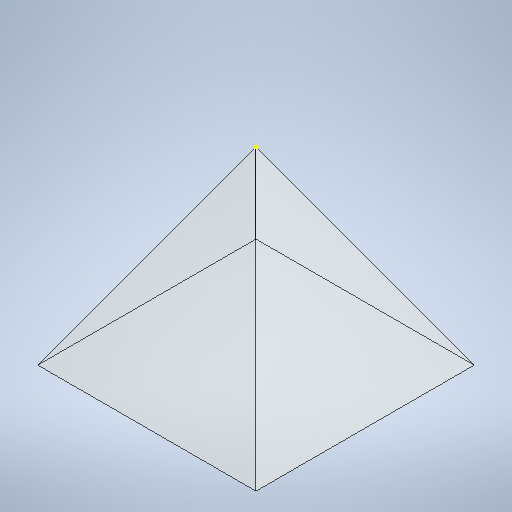
# Autodesk Inventor part: vl53l7cx-FOV
Saved by Autodesk Inventor 2025 (Build 290162000, 162)
## iProperties
Created: 2026-03-19
Part Number: vl53l7cx-FOV
Material: Glass
Document SubType Name: Modeling
Designer: steve
Density: 2.18 g/cm^3
Appearance: Clear
Author: steve
Autodesk Inventor part; units mm, degrees
ref_plane "YZ Plane" through (0, 0, 0) normal (1, 0, 0) x (0, 1, 0)
ref_plane "XZ Plane" through (0, 0, 0) normal (0, 1, 0) x (-1, 0, 0)
sketch "Sketch1" plane through (0, 0, 0) normal (0, 0, 1) x (1, 0, 0)
  line L0 (0, 200) -> (0, -1200) construction
  line L1 (-808.2904, 0) -> (808.2904, 0) construction
  line L2 (0, 0) -> (-577.3503, -1000)
  line L3 (-577.3503, -1000) -> (577.3503, -1000)
  line L4 (577.3503, -1000) -> (0, 0)
  point P0 (0, -1000)
  dimension "d0" = 60
  dimension "d1" = 1000
  constraints: 6 end point, 1 horizontal, 1 midpoint, 1 point on line
  measures "d0" angle of L4 L2
  measures "d1" distance from line of L2.start L3
sketch "Sketch2" plane through (0, 0, 0) normal (1, 0, 0) x (0, 1, 0)
  line L0 (0, 0) -> (-1000, 577.3503)
  line L1 (-1000, 577.3503) -> (-1000, -577.3503)
  line L2 (-1000, -577.3503) -> (0, 0)
  line L3 (0, 677.3503) -> (-1000, 677.3503)
  line L4 (-1000, 677.3503) -> (-1000, -677.3503)
  line L5 (-1000, -677.3503) -> (0, -677.3503)
  line L6 (0, -677.3503) -> (0, 677.3503)
  point P0 (-1000, 0)
  point P1 (-1000, 0)
  point P2 (-1000, 0)
  point P3 (-1000, 0)
  dimension "d2" = 60
  dimension "d4" = 100
  constraints: 14 end point, 2 midpoint, 2 parallel, 1 coincident, 1 collinear, 1 horizontal, 1 perpendicular, 1 vertical
  measures "d2" angle of L2 L0
  measures "d4" distance from line of L3 L0.end
extrude "Extrusion1" add sketch "Sketch1" along normal mid plane 1200
extrude "Extrusion2" cut sketch "Sketch2" along normal mid plane 1200 contours L6 L5 L4 L2 | L0 L4 L3 L6
ref_plane "Work Plane1" through (0, 0, 0) normal (0, -0.5, 0.866) x (1, 0, 0)
sketch "Sketch3" plane through (0, 0, 0) normal (0, -0.5, 0.866) x (1, 0, 0)
  point P0 (0, 0)
body "Solid1"
